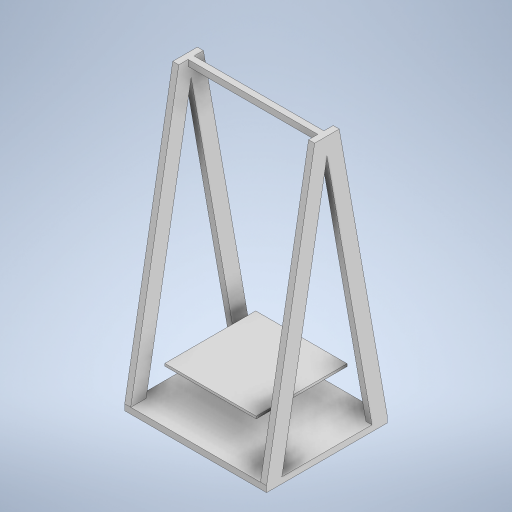
# Autodesk Inventor part: Estructura AA
Saved by Autodesk Inventor 2024 (Build 280153000, 153)
## iProperties
Created: 2024-07-20
Part Number: Estructura AA
Material: Generic
Document SubType Name: Modeling
Designer: compu
Density: 1 g/cm^3
Appearance: Default
Author: compu
Autodesk Inventor part; units mm, degrees
ref_plane "YZ Plane" through (0, 0, 0) normal (1, 0, 0) x (0, 1, 0)
ref_plane "XZ Plane" through (0, 0, 0) normal (0, 1, 0) x (-1, 0, 0)
ref_plane "XY Plane" through (0, 0, 0) normal (0, 0, 1) x (1, 0, 0)
sketch "Sketch1" plane through (0, 0, 0) normal (0, 1, 0) x (-1, 0, 0)
  line L0 (235, -200) -> (-235, -200)
  line L1 (-235, -200) -> (-235, 200)
  line L2 (-235, 200) -> (235, 200)
  line L3 (235, 200) -> (235, -200)
  line L4 (329, 0) -> (-329, 0) projected
  line L5 (0, -280) -> (0, 280) projected
  point P0 (0, 0)
  dimension "d0" = 470
  dimension "d1" = 400
  constraints: 8 end point, 2 parallel, 1 horizontal, 1 perpendicular, 2 other
  measures "d0" distance of L0.start L0.end
  measures "d1" distance of L0.end L1.end
extrude "Extrusion1" add sketch "Sketch1" along normal blind 20
sketch "Sketch2" plane through (0, 20, 0) normal (0, 1, 0) x (1, 0, 0)
  line L0 (-235, -200) -> (235, -200) projected
  line L1 (235, -200) -> (235, 200) projected
  line L2 (235, 200) -> (-235, 200) projected
  line L3 (-235, 200) -> (-235, -200) projected
  line L4 (-329, 0) -> (329, 0) projected
  line L5 (0, 280) -> (0, -280) projected
  circle A0 centre (0, 0) radius 20
  dimension "d4" = 40
  constraints: 1 centre point, 1 coincident
  measures "d4" diameter of A0
extrude "Extrusion2" add sketch "Sketch2" along normal blind 125 contours A0 L4 L5 | L5 L4 A0 | A0 L5 L4 | L5 A0 L4
sketch "Sketch3" plane through (0, 145, 0) normal (0, 1, 0) x (1, 0, 0)
  line L0 (-151.5, 150.5) -> (151.5, 150.5)
  line L1 (151.5, 150.5) -> (151.5, -150.5)
  line L2 (151.5, -150.5) -> (-151.5, -150.5)
  line L3 (-151.5, -150.5) -> (-151.5, 150.5)
  line L4 (-329, 0) -> (329, 0) projected
  line L5 (0, 280) -> (0, -280) projected
  point P0 (0, 0)
  dimension "d7" = 303
  dimension "d8" = 301
  constraints: 8 end point, 2 parallel, 1 horizontal, 1 perpendicular, 2 other
  measures "d7" distance of L1.end L2.end
  measures "d8" distance of L0.end L1.end
extrude "Extrusion3" add sketch "Sketch3" along normal blind 8
ref_plane "Work Plane1" through (0, 903, 0) normal (0, 1, 0) x (1, 0, 0)
sketch "Sketch4" plane through (0, 903, 0) normal (0, 1, 0) x (1, 0, 0)
  line L0 (-235, 10) -> (235, 10)
  line L1 (235, 10) -> (235, -10)
  line L2 (235, -10) -> (-235, -10)
  line L3 (-235, -10) -> (-235, 10)
  circle A0 centre (0, 0) radius 20 projected
  line L4 (-235, -200) -> (235, -200) projected
  line L5 (235, -200) -> (235, 200) projected
  line L6 (235, 200) -> (-235, 200) projected
  line L7 (-235, 200) -> (-235, -200) projected
  line L8 (-329, 0) -> (329, 0) projected
  line L9 (0, 280) -> (0, -280) projected
  dimension "d12" = 20
  constraints: 8 end point, 2 collinear, 2 parallel, 1 horizontal, 1 perpendicular, 1 other
  measures "d12" distance of L0.end L1.end
extrude "Extrusion4" add sketch "Sketch4" along normal blind 20 contours L0 A0 L8 L3 | L0 L9 L8 A0 | L8 A0 L2 L3 | L0 A0 L8 L9 | L8 L9 L2 A0 | L0 L1 L8 A0 | L8 A0 L2 L9 | L8 L1 L2 A0
sketch "Sketch5" plane through (235, 0, 200) normal (1, 0, 0) x (0, 0, -1)
  line L0 (190, 903) -> (210, 903) projected
  line L1 (210, 903) -> (210, 923) projected
  line L2 (190, 923) -> (210, 923) projected
  line L3 (190, 903) -> (190, 923) projected
  line L4 (0, 0) -> (400, 0) projected
  line L5 (0, 20) -> (400, 20) projected
  line L6 (0, 0) -> (0, 20) projected
  line L7 (400, 0) -> (400, 20) projected
  line L8 (0, 0) -> (400, 0) projected
  line L9 (400, 0) -> (400, 20) projected
  line L10 (0, 20) -> (400, 20) projected
  line L11 (0, 0) -> (0, 20) projected
  line L12 (159.2233, 923) -> (240.7767, 923)
  line L13 (0, 20) -> (159.2233, 923)
  line L14 (200, -184.6) -> (200, 1107.6) projected
  line L15 (400, 20) -> (240.7767, 923)
  line L16 (190, 923) -> (210, 923) projected
  line L17 (0, 20) -> (50.7713, 20)
  line L18 (349.2287, 20) -> (400, 20)
  line L19 (349.2287, 20) -> (200, 866.3178)
  line L20 (50.7713, 20) -> (200, 866.3178)
  point P0 (200, 0)
  dimension "d16" = 80
  dimension "d18" = 80
  constraints: 14 end point, 3 collinear, 2 parallel, 2 point on line, 2 symmetric about line, 1 horizontal
  measures "d16" angle of L5 L13
  measures "d18" angle of L5 L15
extrude "Extrusion5" add sketch "Sketch5" against normal blind 20 contours L3 L2 L14 L0 | L0 L14 L20 L5 L13 L12 L3 | L14 L2 L1 L0 | L0 L1 L12 L15 L5 L19 L14
sketch "Sketch6" plane through (-235, 903, -10) normal (-1, 0, 0) x (0, 0, 1)
  line L0 (-40, -60) -> (60, -60) construction
  line L1 (60, -60) -> (60, -188) construction
  line L2 (60, -188) -> (-40, -188) construction
  line L3 (-40, -188) -> (-40, -60) construction
  line L4 (10, -1087.6) -> (10, 204.6) projected
  line L5 (0, 0) -> (20, 0) projected
  line L6 (20, 0) -> (20, 20) projected
  line L7 (0, 20) -> (20, 20) projected
  line L8 (0, 0) -> (0, 20) projected
  line L9 (20, 0) -> (20, 20) projected
  line L10 (0, 0) -> (20, 0) projected
  line L11 (0, 20) -> (0, 0) projected
  line L12 (0, 20) -> (-30.7767, 20) projected
  line L13 (-30.7767, 20) -> (-190, -883) projected
  line L14 (-139.2287, -883) -> (-190, -883) projected
  line L15 (-139.2287, -883) -> (10, -36.6822) projected
  line L16 (10, -36.6822) -> (159.2287, -883) projected
  line L17 (210, -883) -> (159.2287, -883) projected
  line L18 (210, -883) -> (50.7767, 20) projected
  line L19 (50.7767, 20) -> (20, 20) projected
  line L20 (-30.7767, 20) -> (-190, -883) projected
  line L21 (-190, -883) -> (-30.7767, 20)
  line L22 (-30.7767, 20) -> (50.7767, 20)
  line L23 (210, -883) -> (50.7767, 20)
  line L24 (159.2287, -883) -> (210, -883)
  line L25 (159.2287, -883) -> (10, -36.6822)
  line L26 (-139.2287, -883) -> (10, -36.6822) projected
  line L27 (10, -36.6822) -> (-139.2287, -883)
  line L28 (-139.2287, -883) -> (-190, -883)
  point P0 (10, -903)
  dimension "d21" = 100
  dimension "d22" = 128
  dimension "d23" = 60
  constraints: 22 end point, 8 equal length, 2 horizontal, 1 perpendicular, 1 other
  measures "d21" distance of L0.start L0.end
  measures "d22" distance of L0.end L1.end
  measures "d23" distance between parallel lines of L5 L0
extrude "Extrusion6" add sketch "Sketch6" against normal blind 20
body "Solid1"
